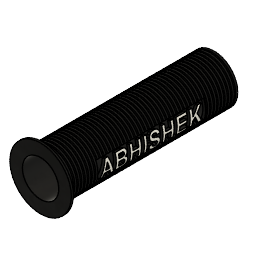
Day 7 Bike Handlebar Grip (Autodesk Fusion 360 design; units mm, degrees)
part number: 2026-07-09-04-35-16-906
Autodesk Fusion 360 part; units mm, degrees
note: some values were not read from the file. Set by a fixed rule: which sketch regions a step uses.
sketch "Sketch1" plane through (0, 0, 0) normal (0, 0, 1) x (1, 0, 0)
  circle A0 centre (0, 0) radius 15
  dimension "d1" = 30
  constraint coincident A0.centre origin
  measures "d1" diameter of A0
extrude "Extrude1" add sketch "Sketch1" along normal blind 125 makes body 1
sketch "Sketch2" plane through (0, 0, 0) normal (1, 0, 0) x (0, 0, -1)
  line L0 (-125, -15) -> (0, -15) construction
  line L1 (0, -15) -> (0, 15) construction
  line L2 (0, 15) -> (-125, 15) construction
  line L3 (-125, 15) -> (-125, -15) construction
  point P0 (-125, -15)
  point P1 (-125, 15)
  point P2 (0, -15)
  point P3 (0, 15)
  dimension "d4" = 10
  text T0 "ABHISHEK " font "Arial" height 10 bold align centre middle in box 125 x 30 at (-125, -15) x (1, 0) y (0, 1) spacing 1
  constraint coincident P0
  constraint coincident P2
  constraint coincident P3
shell "Shell1" thickness 2 removed faces 1 at (3.8315, 5.6199, 125) on bodies 1
emboss "Emboss1" depth 2 profiles "Sketch2" section 1 text T0 onto face at (14.9814, -0.7477, 83.3333) on bodies 1 bodies 1
sketch "Sketch3" plane through (0, 0, 125) normal (0, 0, 1) x (1, 0, 0)
  circle A0 centre (0, 0) radius 15
  circle A1 centre (0, 0) radius 15
  circle A2 centre (0, 0) radius 17
  line L0 (15.4883, 7.0081) -> (13.8704, 5.7106)
  line L1 (15.4913, -7.0014) -> (13.8732, -5.7038)
  circle A3 centre (0, 0) radius 13
  point P0 (16.0643, 5.5623)
  point P1 (16.0643, -5.5623)
  dimension "d10" = 2
  constraint coincident A2 L0.start
  constraint coincident A1 L0.end
  constraint coincident A2 L1.start
  constraint coincident A1 L1.end
extrude "Extrude2" add sketch "Sketch3" against normal blind 1.5 separate body contours A0 A1 A2 L0 L1 | A0 A1 A2 L0 L1 makes body 2
pattern_linear "R-Pattern1" count 50 spacing 2.5 along (0, 0, -1) of bodies 2 makes body 3 at (14.2221, -7.9636, 122.5) makes body 4 at (14.2221, -7.9636, 120) makes body 5 at (14.2221, -7.9636, 117.5) makes body 6 at (14.2221, -7.9636, 115) makes body 7 at (14.2221, -7.9636, 112.5) makes body 8 at (14.2221, -7.9636, 110) makes body 9 at (14.2221, -7.9636, 107.5) makes body 10 at (14.2221, -7.9636, 105) makes body 11 at (14.2221, -7.9636, 102.5) makes body 12 at (14.2221, -7.9636, 100) makes body 13 at (14.2221, -7.9636, 97.5) makes body 14 at (14.2221, -7.9636, 95) makes body 15 at (14.2221, -7.9636, 92.5) makes body 16 at (14.2221, -7.9636, 90) makes body 17 at (14.2221, -7.9636, 87.5) makes body 18 at (14.2221, -7.9636, 85) makes body 19 at (14.2221, -7.9636, 82.5) makes body 20 at (14.2221, -7.9636, 80) makes body 21 at (14.2221, -7.9636, 77.5) makes body 22 at (14.2221, -7.9636, 75) makes body 23 at (14.2221, -7.9636, 72.5) makes body 24 at (14.2221, -7.9636, 70) makes body 25 at (14.2221, -7.9636, 67.5) makes body 26 at (14.2221, -7.9636, 65) makes body 27 at (14.2221, -7.9636, 62.5) makes body 28 at (14.2221, -7.9636, 60) makes body 29 at (14.2221, -7.9636, 57.5) makes body 30 at (14.2221, -7.9636, 55) makes body 31 at (14.2221, -7.9636, 52.5) makes body 32 at (14.2221, -7.9636, 50) makes body 33 at (14.2221, -7.9636, 47.5) makes body 34 at (14.2221, -7.9636, 45) makes body 35 at (14.2221, -7.9636, 42.5) makes body 36 at (14.2221, -7.9636, 40) makes body 37 at (14.2221, -7.9636, 37.5) makes body 38 at (14.2221, -7.9636, 35) makes body 39 at (14.2221, -7.9636, 32.5) makes body 40 at (14.2221, -7.9636, 30) makes body 41 at (14.2221, -7.9636, 27.5) makes body 42 at (14.2221, -7.9636, 25) makes body 43 at (14.2221, -7.9636, 22.5) makes body 44 at (14.2221, -7.9636, 20) makes body 45 at (14.2221, -7.9636, 17.5) makes body 46 at (14.2221, -7.9636, 15) makes body 47 at (14.2221, -7.9636, 12.5) makes body 48 at (14.2221, -7.9636, 10) makes body 49 at (14.2221, -7.9636, 7.5) makes body 50 at (14.2221, -7.9636, 5) makes body 51 at (14.2221, -7.9636, 2.5)
extrude "Extrude3" cut sketch "Sketch3" against normal blind 77 from surface at -24 contours A0 A1 A2 L0 L1 picked at (15.227, 5.8234) bodies 12 13 14 15 16 17 18 19 20 21 22 23 24 25 26 27 28 29 30 31 32 33 34 35 36 37 38 39 40 41 42
combine "Combine1" operation add target body 1 tool bodies 2 41 20 22 21 24 23 17 18 19 7 8 49 47 48 44 46 42 43 45 16 9 10 11 13 14 12 15 28 29 26 30 27 25 50 51 32 36 33 34 31 35 37 5 3 6 4 39 40 38
sketch "Sketch4" plane through (0, 0, 125) normal (0, 0, 1) x (1, 0, 0)
  circle A0 centre (0, 0) radius 17
  circle A1 centre (0, 0) radius 13
  circle A2 centre (0, 0) radius 17
  circle A3 centre (0, 0) radius 22
  dimension "d21" = 5
extrude "Extrude4" add sketch "Sketch4" against normal blind 1.5 contours A3 bodies 1
equation "d5 = 'ABHISHEK '"
